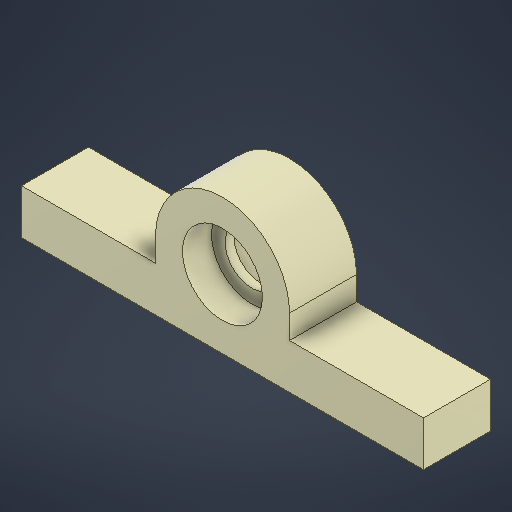
# Autodesk Inventor part: wheel_bearing_no_flange
Saved by Autodesk Inventor 2026 (Build 300175050, 175E)
## iProperties
Created: 2025-06-04
Part Number: wheel_bearing_no_flange
Material: Generic
Document SubType Name: Modeling
Designer: satom
Density: 1 g/cm^3
Appearance: Smooth - Ash
Author: satom
Autodesk Inventor part; units mm, degrees
ref_plane "YZ Plane" through (0, 0, 0) normal (1, 0, 0) x (0, 1, 0)
ref_plane "XZ Plane" through (0, 0, 0) normal (0, 1, 0) x (-1, 0, 0)
ref_plane "XY Plane" through (0, 0, 0) normal (0, 0, 1) x (1, 0, 0)
sketch "Sketch1" plane through (0, 0, 0) normal (0, 0, 1) x (1, 0, 0)
  line L0 (0, 0) -> (76.2, 0)
  line L1 (50.8, 8.5) -> (50.8, 13)
  line L2 (25.4, 8.5) -> (25.4, 13)
  arc A0 (50.8, 13) -> (25.4, 13) centre (38.1, 13) ccw
  line L3 (0, 8.5) -> (25.4, 8.5)
  line L4 (76.2, 8.5) -> (50.8, 8.5)
  line L5 (76.2, 8.5) -> (76.2, 0)
  line L6 (0, 8.5) -> (0, 0)
  dimension "d0" = 76.2
  dimension "d4" = 25.4
  dimension "d18" = 13
  dimension "d20" = 25.4
  dimension "d21" = 8.5
  dimension "d22" = 8.5
  dimension "d23" = 12.7
  dimension "d24" = 25.4
  dimension "d25" = 12.7
  constraints: 14 end point, 2 point on circle, 2 point on line, 2 vertical, 1 centre point, 1 horizontal, 1 perpendicular
  measures "d0" distance of L0.start L0.end
  measures "d4" distance between parallel lines of L1 L2
  measures "d18" distance from line of L0 A0.centre
  measures "d20" distance of L4.start L1.start
  measures "d21" distance of L3.start L0.start
  measures "d22" distance of L4.start L0.end
  measures "d23" radius of A0
  measures "d24" distance of L3.start L2.start
  measures "d25" horizontal distance of L2.start A0.centre
extrude "BearingBlock" add sketch "Sketch1" along normal blind 12.7
sketch "Sketch2" plane through (0, 0, 12.7) normal (0, 0, 1) x (1, 0, 0)
  arc A0 (50.8, 13) -> (25.4, 13) centre (38.1, 13) ccw projected
  line L0 (0, 0) -> (76.2, 0) projected
  circle A1 centre (38.1, 13) radius 7.575
  point P0 (38.1, 25.7)
  dimension "d8" = 15.15
  dimension "d26" = 13
  constraints: 1 centre point, 1 coincident, 1 point on circle
  measures "d8" diameter of A1
  measures "d26" distance from line of L0 A0.centre
extrude "BearingMount" cut sketch "Sketch2" against normal blind 5.5
sketch "Sketch4" plane through (0, 0, 0) normal (0, 0, -1) x (-1, 0, 0)
  circle A0 centre (-38.1, 13) radius 7.575 projected
  circle A1 centre (-38.1, 13) radius 7.575
  line L0 (0, 0) -> (-76.2, 0) projected
  dimension "d27" = 15.15
  dimension "d28" = 13
  constraints: 1 centre point, 1 coincident
  measures "d27" diameter of A0
  measures "d28" distance from line of L0 A1.centre
extrude "BearingMount2" cut sketch "Sketch4" against normal blind 5.5
sketch "Sketch3" plane through (0, 0, 0) normal (0, -1, 0) x (1, 0, 0)
  line L0 (0, 0) -> (0, 12.7) projected
  line L1 (-76.2, 6.35) -> (76.2, 6.35) construction
  line L2 (76.2, 0) -> (76.2, 12.7) projected
  circle A0 centre (12.7, 6.35) radius 2
  circle A1 centre (63.5, 6.35) radius 2
  point P0 (0, 6.35)
  dimension "d11" = 12.7
  dimension "d12" = 12.7
  dimension "d13" = 4
  dimension "d14" = 4
  dimension "d15" = 50.8
  constraints: 3 midpoint, 2 centre point, 2 end point, 2 point on line
  measures "d11" distance from line of L0 A0.centre
  measures "d12" distance from line of L2 A1.centre
  measures "d13" diameter of A1
  measures "d14" diameter of A0
  measures "d15" distance of A0.centre A1.centre
extrude "HeatSetInsert" cut sketch "Sketch3" against normal blind 7
sketch "Sketch5" plane through (38.1, 13, 5.5) normal (0, 0, -1) x (-1, 0, 0)
  circle A0 centre (0, 0) radius 7.575 projected
  circle A1 centre (0, 0) radius 5
  line L0 (38.1, -13) -> (-38.1, -13) projected
  dimension "d32" = 10
  dimension "d33" = 13
  constraints: 1 centre point, 1 coincident
  measures "d32" diameter of A1
  measures "d33" distance from line of L0 A1.centre
extrude "Extrusion5" cut sketch "Sketch5" against normal through all contours A1
equation "\"d18\" = motor_centerline_height"
equation "\"d13\" = m3_heat_set_insert"
equation "\"d14\" = m3_heat_set_insert"
equation "\"m3_heat_set_insert\" = 4"
equation "\"m3_clearance\" = 3.4"
equation "\"m3_heat_set_depth\" = 7"
equation "\"robot_diameter\" = 354"
equation "\"hardboard_thickness\" = 5"
equation "\"motor_centerline_height\" = 13"
body "Solid1"
